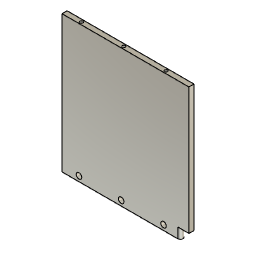
side_cover_side_wall v31 (Autodesk Fusion 360 design; units mm, degrees)
Autodesk Fusion 360 part; units mm, degrees
note: some values were not read from the file. Chosen so that the rebuilt part matches the saved one: which bodies a step acts on; which face or edge a step refers to; how an offset face is resized; which pieces of a blend or face edit are solid.
sketch "Sketch1" plane through (0, 0, 0) normal (0, 0, 1) x (1, 0, 0)
  line L0 (0, 0) -> (150, 0)
  line L1 (150, 0) -> (150, 10)
  line L2 (150, 10) -> (0, 10)
  line L3 (0, 10) -> (0, 0)
  dimension "d1" = 150
  dimension "d2" = 10
  constraint horizontal L0
  constraint vertical L1
  constraint horizontal L2
  constraint vertical L3
  constraint coincident L0.start L3.end
  measures "d1" distance of L0.start L0.end
  measures "d2" distance of L0.start L2.end
extrude "Extrude1" add sketch "Sketch1" along normal blind 137.719 makes body 1
sketch "Sketch2" plane through (0, 0, 137.719) normal (0, 0, 1) x (-1, 0, 0)
  line L0 (0, -10) -> (0, 0)
  line L1 (0, 0) -> (-150, 0)
  line L2 (-150, 0) -> (-150, -10)
  line L3 (-150, -10) -> (0, -10)
  line L4 (0, -5) -> (-25, -5)
  line L5 (-150, -5) -> (-125, -5)
  dimension "d5" = 25
  dimension "d6" = 25
  constraint midpoint L0 L4.start
  constraint perpendicular L0 L4
  constraint midpoint L2 L5.start
  constraint perpendicular L2 L5
  measures "d5" distance of L4.start L4.end
  measures "d6" distance of L5.start L5.end
sketch "Sketch3" plane through (0, 0, 0) normal (-1, 0, 0) x (0, -1, 0)
  line L0 (-10, 0) -> (0, 0)
  line L1 (0, 0) -> (0, 137.719)
  line L2 (0, 137.719) -> (-10, 137.719)
  line L3 (-10, 137.719) -> (-10, 0)
  line L4 (-5, 0) -> (-5, 25)
  line L5 (-5, 137.719) -> (-5, 112.719)
  dimension "d10" = 25
  dimension "d11" = 25
  constraint parallel L3 L4
  constraint midpoint L2 L5.start
  constraint perpendicular L2 L5
  measures "d10" distance of L4.start L4.end
  measures "d11" distance of L5.start L5.end
extrude "Extrude2" cut 1 faces at (100, 10, 45.9063) along direction (0, -1, 0) blind 4 on bodies 1 bodies 1
sketch "Sketch4" plane through (0, 0, 137.719) normal (0, 0, 1) x (-1, 0, 0)
  line L0 (-150, -6) -> (0, -6)
  line L1 (0, -6) -> (0, 0)
  line L2 (0, 0) -> (-150, 0)
  line L3 (-150, 0) -> (-150, -6)
  line L4 (0, -3) -> (-31, -3)
  line L5 (-150, -3) -> (-125, -3)
  dimension "d17" = 31
  dimension "d18" = 25
  constraint midpoint L1 L4.start
  constraint perpendicular L1 L4
  constraint midpoint L3 L5.start
  constraint perpendicular L3 L5
  measures "d17" distance of L4.start L4.end
  measures "d18" distance of L5.start L5.end
sketch "Sketch5" plane through (0, 0, 0) normal (-1, 0, 0) x (0, -1, 0)
  line L0 (-6, 137.719) -> (-6, 0)
  line L1 (-6, 0) -> (0, 0)
  line L2 (0, 0) -> (0, 137.719)
  line L3 (0, 137.719) -> (-6, 137.719)
  line L4 (-3, 137.719) -> (-3, 112.719)
  line L5 (-3, 0) -> (-3, 25)
  dimension "d22" = 25
  dimension "d23" = 25
  constraint midpoint L3 L4.start
  constraint perpendicular L3 L4
  constraint midpoint L1 L5.start
  constraint perpendicular L1 L5
  measures "d22" distance of L4.start L4.end
  measures "d23" distance of L5.start L5.end
hole "Hole4" at (0, 3, 112.719) at (0, 3, 25) direction (1, 0, 0) diameter 3.529 depth 10 tip angle 180 bodies 1
thread "Thread4" "ISO Metric profile 4.0 M4x0.5 6H"
sketch "Sketch6" plane through (0, 0, 137.719) normal (0, 0, 1) x (-1, 0, 0)
  line L0 (-150, -6) -> (0, -6)
  line L1 (0, -6) -> (0, 0)
  line L2 (0, 0) -> (-150, 0)
  line L3 (-150, 0) -> (-150, -6)
  line L4 (0, -3) -> (-25, -3)
  dimension "d27" = 25
  constraint midpoint L1 L4.start
  constraint perpendicular L1 L4
  measures "d27" distance of L4.start L4.end
extrude "Extrude3" cut 1 faces at (50, 4, 0) along direction (0, 0, 1) blind 4 on bodies 1 bodies 1
extrude "Extrude4" cut 1 faces at (50, 4, 4) along direction (0, 0, 1) blind 1 on bodies 1 bodies 1
sketch "Sketch7" plane through (0, 0, 5) normal (0, 0, -1) x (1, 0, 0)
  line L0 (0, -6) -> (150, -6)
  line L1 (150, -6) -> (150, 0)
  line L2 (150, 0) -> (0, 0)
  line L3 (0, 0) -> (0, -6)
  line L4 (0, -3) -> (25, -3)
  line L5 (150, -3) -> (125, -3)
  dimension "d35" = 25
  dimension "d36" = 25
  constraint midpoint L3 L4.start
  constraint perpendicular L3 L4
  constraint midpoint L1 L5.start
  constraint perpendicular L1 L5
  measures "d35" distance of L4.start L4.end
  measures "d36" distance of L5.start L5.end
sketch "Sketch8" plane through (0, 0, 0) normal (-1, 0, 0) x (0, -1, 0)
  circle A0 centre (-3, 112.719) radius 1.7644
  circle A1 centre (-3, 25) radius 1.7644
  line L0 (-6, 5) -> (0, 5)
  line L1 (0, 5) -> (0, 137.719)
  line L2 (0, 137.719) -> (-6, 137.719)
  line L3 (-6, 137.719) -> (-6, 5)
  line L4 (-3, 5) -> (-3, 30)
  dimension "d40" = 25
  constraint midpoint L0 L4.start
  constraint perpendicular L0 L4
  measures "d40" distance of L4.start L4.end
hole "Hole7" at (0, 3, 30) direction (1, 0, 0) diameter 3.332 depth 10 tip angle 180 bodies 1
thread "Thread7" "ISO Metric profile 4.0 M4x0.5 6H" major diameter 4.0861 minor diameter 3.5287 pitch 0.5 angle 60 resizes the face on face at (3.3333, 3.083, 31.6639) on bodies 1
delete_face "DeleteFace2" 2 faces at (6.6667, 3.1757, 26.7557) (10, 3.2552, 25.5942) on bodies 1
sketch "Sketch9" plane through (0, 0, 0) normal (0, -1, 0) x (1, 0, 0)
  line L0 (0, 5) -> (150, 5)
  line L1 (150, 5) -> (150, 137.719)
  line L2 (150, 137.719) -> (0, 137.719)
  line L3 (0, 137.719) -> (0, 5)
  line L4 (150, 5) -> (130, 5)
  line L5 (130, 5) -> (130, 11)
  line L6 (130, 11) -> (150, 11)
  line L7 (150, 11) -> (150, 5)
  line L8 (130, 11) -> (72, 11)
  line L9 (0, 5) -> (20, 5)
  line L10 (20, 5) -> (20, 11)
  line L11 (20, 11) -> (0, 11)
  line L12 (0, 11) -> (0, 5)
  dimension "d44" = 20
  dimension "d45" = 6
  dimension "d46" = 58
  dimension "d47" = 20
  dimension "d48" = 6
  constraint horizontal L4
  constraint vertical L5
  constraint horizontal L6
  constraint vertical L7
  constraint coincident L0.end L1.start
  constraint perpendicular L5 L8
  constraint horizontal L9
  constraint vertical L10
  constraint horizontal L11
  constraint vertical L12
  constraint coincident L0.start L3.end
  measures "d44" distance of L0.end L4.end
  measures "d45" distance of L0.end L6.end
  measures "d46" distance of L5.end L8.end
  measures "d47" distance of L0.start L9.end
  measures "d48" distance of L0.start L11.end
hole "Hole8" at (20, 0, 11) at (72, 0, 11) at (130, 0, 11) direction (0, 1, 0) diameter 6.6 depth 20 tip angle 180 bodies 1
extrude "Extrude5" add 1 faces at (50, 4, 137.719) along direction (0, 0, 1) blind 12 on bodies 1 bodies 1
delete_face "DeleteFace3" 1 faces at (6.6667, 3.1757, 31.7556) on bodies 1
delete_face "DeleteFace4" 1 faces at (6.6667, 2.1561, 114.2686) on bodies 1
extrude "Extrude6" add 1 faces at (50, 4, 149.719) along direction (0, 0, 1) blind 13 on bodies 1 bodies 1
sketch "Sketch10" plane through (0, 0, 0) normal (-1, 0, 0) x (0, -1, 0)
  line L0 (-6, 5) -> (0, 5)
  line L1 (0, 5) -> (0, 162.719)
  line L2 (0, 162.719) -> (-6, 162.719)
  line L3 (-6, 162.719) -> (-6, 5)
  line L4 (-3, 5) -> (-3, 25)
  line L5 (-3, 162.719) -> (-3, 142.719)
  dimension "d56" = 20
  dimension "d57" = 20
  constraint midpoint L0 L4.start
  constraint perpendicular L0 L4
  constraint midpoint L2 L5.start
  constraint perpendicular L2 L5
  measures "d56" distance of L4.start L4.end
  measures "d57" distance of L5.start L5.end
hole "Hole9" at (0, 3, 142.719) at (0, 3, 25) direction (1, 0, 0) diameter 3.332 depth 10 tip angle 180 bodies 1
thread "Thread8" "ISO Metric profile 4.0 M4x0.5 6H" major diameter 4.0861 minor diameter 3.5287 pitch 0.5 angle 60 resizes the face on face at (3.3333, 1.3963, 143.1702) on face at (3.3333, 3.083, 26.6639) on bodies 1
delete_face "DeleteFace5" 1 faces at (72.6539, 2, 7.7654) on bodies 1
sketch "Sketch11" plane through (0, 0, 0) normal (0, -1, 0) x (1, 0, 0)
  circle A0 centre (20, 11) radius 3.3
  circle A1 centre (130, 11) radius 3.3
  line L0 (0, 5) -> (150, 5)
  line L1 (150, 5) -> (150, 162.719)
  line L2 (150, 162.719) -> (0, 162.719)
  line L3 (0, 162.719) -> (0, 5)
  line L4 (20, 11) -> (76, 11)
  dimension "d61" = 56
  constraint coincident A0.centre L4.start
  constraint horizontal L4
  measures "d61" distance of A0.centre L4.end
hole "Hole10" at (76, 0, 11) direction (0, 1, 0) diameter 6.6 depth 10 tip angle 180 bodies 1
sketch "Sketch12" plane through (0, 0, 162.719) normal (0, 0, 1) x (-1, 0, 0)
  line L0 (-150, -6) -> (0, -6)
  line L1 (0, -6) -> (0, 0)
  line L2 (0, 0) -> (-150, 0)
  line L3 (-150, 0) -> (-150, -6)
  line L4 (0, -3) -> (-20, -3)
  line L5 (-20, -3) -> (-75, -3)
  line L6 (-150, -3) -> (-130, -3)
  dimension "d65" = 20
  dimension "d66" = 55
  dimension "d67" = 20
  constraint midpoint L1 L4.start
  constraint perpendicular L1 L4
  constraint horizontal L5
  constraint midpoint L3 L6.start
  constraint perpendicular L3 L6
  measures "d65" distance of L4.start L4.end
  measures "d66" distance of L4.end L5.end
  measures "d67" distance of L6.start L6.end
hole "Hole11" at (20, 3, 162.719) at (75, 3, 162.719) at (130, 3, 162.719) direction (0, 0, -1) diameter 3.332 depth 10 tip angle 180 bodies 1
thread "Thread9" "ISO Metric profile 4.0 M4x0.5 6H" major diameter 4.0861 minor diameter 3.5287 pitch 0.5 angle 60 resizes the face on face at (20.083, 1.3361, 159.3857) on face at (76.0709, 4.2762, 159.3857) on face at (130.083, 1.3361, 159.3857) on bodies 1
delete_face "DeleteFace6" 1 faces at (76.6539, 2, 7.7654) on bodies 1
sketch "Sketch13" plane through (0, 0, 0) normal (0, -1, 0) x (1, 0, 0)
  circle A0 centre (20, 11) radius 3.3
  circle A1 centre (130, 11) radius 3.3
  line L0 (0, 5) -> (150, 5)
  line L1 (150, 5) -> (150, 162.719)
  line L2 (150, 162.719) -> (0, 162.719)
  line L3 (0, 162.719) -> (0, 5)
  line L4 (20, 11) -> (75, 11)
  dimension "d71" = 55
  constraint coincident A0.centre L4.start
  constraint parallel L0 L4
  measures "d71" distance of A0.centre L4.end
hole "Hole12" at (75, 0, 11) direction (0, 1, 0) diameter 6.6 depth 10 tip angle 180 bodies 1
sketch "Sketch14" plane through (0, 0, 0) normal (-1, 0, 0) x (0, -1, 0)
  circle A0 centre (-3, 142.719) radius 1.7644
  circle A1 centre (-3, 25) radius 1.7644
  line L0 (-6, 5) -> (0, 5)
  line L1 (0, 5) -> (0, 162.719)
  line L2 (0, 162.719) -> (-6, 162.719)
  line L3 (-6, 162.719) -> (-6, 5)
  line L4 (-3, 142.719) -> (-3, 122.719)
  line L5 (-3, 25) -> (-3, 45)
  dimension "d75" = 20
  dimension "d76" = 20
  constraint coincident A0.centre L4.start
  constraint parallel L3 L4
  constraint coincident A1.centre L5.start
  constraint parallel L1 L5
  measures "d75" distance of A0.centre L4.end
  measures "d76" distance of A1.centre L5.end
hole "Hole13" at (0, 3, 122.719) at (0, 3, 45) direction (1, 0, 0) diameter 3.332 depth 10 tip angle 180 bodies 1
thread "Thread10" "ISO Metric profile 4.0 M4x0.5 6H" major diameter 4.0861 minor diameter 3.5287 pitch 0.5 angle 60 resizes the face on face at (3.3333, 1.3345, 122.6775) on face at (3.3333, 3.083, 46.6639) on bodies 1
delete_face "DeleteFace7" 2 faces at (6.6667, 3.1757, 26.7556) (10, 3.9224, 25.3119) on bodies 1
delete_face "DeleteFace8" 1 faces at (6.6667, 1.5675, 143.7489) on bodies 1
delete_face "DeleteFace9" 1 faces at (20.1645, 2, 7.7041) on bodies 1
delete_face "DeleteFace10" 1 faces at (75.6539, 2, 7.7654) on bodies 1
delete_face "DeleteFace11" 1 faces at (128.4218, 2, 13.8981) on bodies 1
sketch "Sketch15" plane through (0, 0, 0) normal (0, -1, 0) x (1, 0, 0)
  line L0 (0, 5) -> (150, 5)
  line L1 (150, 5) -> (150, 162.719)
  line L2 (150, 162.719) -> (0, 162.719)
  line L3 (0, 162.719) -> (0, 5)
  line L4 (0, 5) -> (20, 5)
  line L5 (20, 5) -> (20, 11)
  line L6 (20, 11) -> (0, 11)
  line L7 (0, 11) -> (0, 5)
  line L8 (20, 11) -> (70, 11)
  line L9 (70, 11) -> (120, 11)
  dimension "d80" = 20
  dimension "d81" = 6
  dimension "d82" = 50
  dimension "d83" = 50
  constraint horizontal L4
  constraint vertical L5
  constraint horizontal L6
  constraint vertical L7
  constraint coincident L0.start L3.end
  constraint perpendicular L5 L8
  constraint parallel L8 L9
  measures "d80" distance of L0.start L4.end
  measures "d81" distance of L0.start L6.end
  measures "d82" distance of L5.end L8.end
  measures "d83" distance of L8.end L9.end
hole "Hole14" at (20, 0, 11) at (120, 0, 11) at (70, 0, 11) direction (0, 1, 0) diameter 6.6 depth 20 tip angle 180 bodies 1
sketch "Sketch16" plane through (0, 0, 0) normal (0, -1, 0) x (1, 0, 0)
  circle A0 centre (120, 11) radius 3.3
  circle A1 centre (20, 11) radius 3.3
  circle A2 centre (70, 11) radius 3.3
  line L0 (0, 5) -> (150, 5)
  line L1 (150, 5) -> (150, 162.719)
  line L2 (150, 162.719) -> (0, 162.719)
  line L3 (0, 162.719) -> (0, 5)
  line L4 (150, 5) -> (140, 5)
  line L5 (140, 5) -> (140, 17)
  line L6 (140, 17) -> (150, 17)
  line L7 (150, 17) -> (150, 5)
  dimension "d87" = 10
  dimension "d88" = 12
  constraint horizontal L4
  constraint vertical L5
  constraint horizontal L6
  constraint vertical L7
  constraint coincident L0.end L1.start
  measures "d87" distance of L0.end L4.end
  measures "d88" distance of L0.end L6.end
extrude "Extrude7" cut sketch "Sketch16" against normal blind 15 contours L0 L1 L4 L5 L6 L7 bodies 1
sketch "Sketch17" plane through (0, 0, 5) normal (0, 0, -1) x (1, 0, 0)
  line L0 (140, -6) -> (140, 0)
  line L1 (140, 0) -> (0, 0)
  line L2 (0, 0) -> (0, -6)
  line L3 (0, -6) -> (140, -6)
  line L4 (140, -6) -> (137, -6)
  line L5 (137, -6) -> (137, -3)
  line L6 (137, -3) -> (140, -3)
  line L7 (140, -3) -> (140, -6)
  circle A0 centre (137, -3) radius 3
  dimension "d91" = 3
  dimension "d92" = 3
  dimension "d93" = 6
  constraint horizontal L4
  constraint vertical L5
  constraint horizontal L6
  constraint vertical L7
  constraint coincident L0.start L3.end
  constraint coincident L5.end L6.start
  measures "d91" distance of L0.start L4.end
  measures "d92" distance of L0.start L6.end
  measures "d93" diameter of A0
extrude "Extrude8" cut sketch "Sketch17" against normal blind 12 contours L0 L3 L4 L7 A0 bodies 1
sketch "Sketch18" plane through (0, 0, 5) normal (0, 0, -1) x (1, 0, 0)
  arc A0 (137, -6) -> (140, -3) centre (137, -3) ccw
  line L0 (140, -3) -> (140, 0)
  line L1 (140, 0) -> (0, 0)
  line L2 (0, 0) -> (0, -6)
  line L3 (0, -6) -> (137, -6)
  circle A1 centre (137, -3) radius 3
  dimension "d96" = 6
  constraint concentric A0 A1
  measures "d96" diameter of A1
extrude "Extrude9" cut sketch "Sketch18" against normal blind 12 contours L0 L1 A1 bodies 1
sketch "Sketch19" plane through (0, 0, 162.719) normal (0, 0, 1) x (-1, 0, 0)
  circle A0 centre (-75, -3) radius 1.7644
  circle A1 centre (-20, -3) radius 1.7644
  circle A2 centre (-130, -3) radius 1.7644
  line L0 (-150, -6) -> (0, -6)
  line L1 (0, -6) -> (0, 0)
  line L2 (0, 0) -> (-150, 0)
  line L3 (-150, 0) -> (-150, -6)
  line L4 (-20, -3) -> (-70, -3)
  line L5 (-70, -3) -> (-120, -3)
  dimension "d99" = 50
  dimension "d100" = 50
  constraint coincident A1.centre L4.start
  constraint parallel L2 L4
  constraint parallel L4 L5
  measures "d99" distance of A1.centre L4.end
  measures "d100" distance of L4.end L5.end
delete_face "DeleteFace12" 2 faces at (74.5646, 1.2902, 159.3857) (74.4907, 2.9677, 152.719) on bodies 1
delete_face "DeleteFace13" 2 faces at (130.4354, 1.2902, 156.0523) (130.9475, 2.4829, 152.719) on bodies 1
hole "Hole15" at (70, 3, 162.719) at (120, 3, 162.719) direction (0, 0, -1) diameter 3.332 depth 10 tip angle 180 bodies 1
thread "Thread11" "ISO Metric profile 4.0 M4x0.5 6H" major diameter 4.0861 minor diameter 3.5287 pitch 0.5 angle 60 resizes the face on face at (71.0709, 4.2762, 159.3857) on face at (121.0709, 4.2762, 159.3857) on bodies 1
ref_plane "WorkPlane1" through (75, 3, 102.719) normal (0, 0, 1) x (1, 0, 0)
split "Split1" by plane through (75, 3, 102.719) normal (0, 0, 1) bodies 1 makes body 2 at (100, 6, 122.719)
move_body "Move1" bodies 2 to x (1, 0, 0) y (0, 1, 0) z (0, 0, 1) at (0, 0, 4.218)
extrude "Extrude10" add 1 faces at (50, 4, 102.719) along direction (0, 0, 1) blind 4.218 on bodies 1 bodies 1 2
split "Split2" by plane through (75, 3, 102.719) normal (0, 0, 1) bodies 1 makes body 3 at (100, 6, 145.531)
move_body "Move2" bodies 3 to x (1, 0, 0) y (0, 1, 0) z (0, 0, 1) at (0, 0, 0.063)
extrude "Extrude11" add 1 faces at (50, 4, 102.719) along direction (0, 0, 1) blind 0.063 on bodies 1 bodies 1 3
